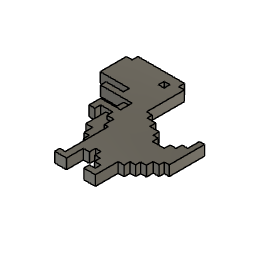
dino (Autodesk Fusion 360 design; units mm, degrees)
Autodesk Fusion 360 part; units mm, degrees
sketch "Dino" plane through (0, 0, 0) normal (0, 0, 1) x (1, 0, 0)
  line L0 (16.5, 0) -> (20, 0)
  line L1 (20, 0) -> (20, 5)
  line L2 (20, 5) -> (21.8166, 5)
  line L3 (21.8166, 5) -> (21.8166, 6.8132)
  line L4 (21.8166, 6.8132) -> (23.4038, 6.8132)
  line L5 (23.4038, 6.8132) -> (23.4038, 5)
  line L6 (23.4038, 5) -> (25, 5)
  line L7 (25, 5) -> (25, 3.315)
  line L8 (25, 3.315) -> (26.8534, 3.315)
  line L9 (26.8534, 3.315) -> (26.8534, 1.6631)
  line L10 (26.8534, 1.6631) -> (25.1529, 1.6631)
  line L11 (25.1529, 1.6631) -> (25.1529, 0)
  line L12 (25.1529, 0) -> (28.5781, 0)
  line L13 (28.5781, 0) -> (28.5781, 6.758)
  line L14 (28.5781, 6.758) -> (30.3565, 6.758)
  line L15 (30.3565, 6.758) -> (30.3565, 8.5127)
  line L16 (30.3565, 8.5127) -> (32, 8.5127)
  line L17 (32, 8.5127) -> (32, 10)
  line L18 (32, 10) -> (33.7351, 10)
  line L19 (33.7351, 10) -> (33.7351, 12)
  line L20 (33.7351, 12) -> (35.5, 12)
  line L21 (35.5, 12) -> (35.5, 13.5)
  line L22 (35.5, 13.5) -> (37, 13.5)
  line L23 (37, 13.5) -> (37, 24)
  line L24 (37, 24) -> (35.5, 24)
  line L25 (35.5, 24) -> (35.5, 20.5)
  line L26 (35.5, 20.5) -> (33.7869, 20.5)
  line L27 (33.7869, 20.5) -> (33.7869, 18.75)
  line L28 (33.7869, 18.75) -> (32, 18.75)
  line L29 (32, 18.75) -> (32, 17.0258)
  line L30 (32, 17.0258) -> (28.5, 17.0258)
  line L31 (28.5, 17.0258) -> (28.5, 18.75)
  line L32 (28.5, 18.75) -> (27, 18.75)
  line L33 (27, 18.75) -> (27, 20.5)
  line L34 (27, 20.5) -> (24.2282, 20.5)
  line L35 (24.2282, 20.5) -> (24.2282, 22.2618)
  line L36 (24.2282, 22.2618) -> (21.6914, 22.2618)
  line L37 (21.6914, 22.2618) -> (21.6914, 23.7839)
  line L38 (21.6914, 23.7839) -> (20, 23.7839)
  line L39 (20, 23.7839) -> (20, 35)
  line L40 (20, 35) -> (18.3225, 35)
  line L41 (18.3225, 35) -> (18.3225, 36.7116)
  line L42 (18.3225, 36.7116) -> (4.5, 36.7116)
  line L43 (4.5, 36.7116) -> (4.5, 35)
  line L44 (4.5, 35) -> (2.7971, 35)
  line L45 (2.7971, 35) -> (2.7971, 27.2137)
  line L46 (2.7971, 27.2137) -> (11.4112, 27.2137)
  line L47 (11.4112, 27.2137) -> (11.4112, 25.5)
  line L48 (11.4112, 25.5) -> (6.2675, 25.5)
  line L49 (6.2675, 25.5) -> (6.2675, 23.8448)
  line L50 (6.2675, 23.8448) -> (13.127, 23.8448)
  line L51 (13.127, 23.8448) -> (13.127, 20.4572)
  line L52 (13.127, 20.4572) -> (9.6973, 20.4572)
  line L53 (9.6973, 20.4572) -> (9.6973, 17)
  line L54 (9.6973, 17) -> (11.4121, 17)
  line L55 (11.4121, 17) -> (11.4121, 18.7286)
  line L56 (11.4121, 18.7286) -> (13, 18.7286)
  line L57 (13, 18.7286) -> (13, 12.7374)
  line L58 (13, 12.7374) -> (15, 12.7374)
  line L59 (15, 12.7374) -> (15, 10.206)
  line L60 (15, 10.206) -> (16.5, 10.206)
  line L61 (16.5, 10.206) -> (16.5, 8.5)
  line L62 (16.5, 8.5) -> (18.1296, 8.5)
  line L63 (18.1296, 8.5) -> (18.1296, 1.5)
  line L64 (18.1296, 1.5) -> (16.5, 1.5)
  line L65 (16.5, 1.5) -> (16.5, 0)
  line L66 (13.127, 23.8448) -> (15.6157, 23.8448)
  line L67 (15.6157, 23.8448) -> (15.6157, 20.4572)
  line L68 (15.6157, 20.4572) -> (13.127, 20.4572)
  line L69 (13, 18.7286) -> (15, 18.7286)
  line L70 (15, 18.7286) -> (15, 17)
  line L71 (15, 17) -> (17, 17)
  line L72 (17, 17) -> (17, 14.1994)
  line L73 (17, 14.1994) -> (18.1296, 14.1994)
  line L74 (18.1296, 14.1994) -> (18.1296, 8.5)
  line L75 (14.802, 34.2204) -> (14.802, 32.5)
  line L76 (14.802, 32.5) -> (16.5, 32.5)
  line L77 (16.5, 32.5) -> (16.5, 34.2204)
  line L78 (16.5, 34.2204) -> (14.802, 34.2204)
  constraint horizontal L0
  constraint perpendicular L0 L1
  constraint perpendicular L1 L2
  constraint perpendicular L0 L3
  constraint perpendicular L3 L4
  constraint perpendicular L0 L5
  constraint perpendicular L3 L6
  constraint perpendicular L0 L7
  constraint perpendicular L7 L8
  constraint perpendicular L8 L9
  constraint perpendicular L9 L10
  constraint perpendicular L8 L11
  constraint perpendicular L9 L12
  constraint perpendicular L12 L13
  constraint perpendicular L13 L14
  constraint perpendicular L14 L15
  constraint perpendicular L15 L16
  constraint perpendicular L16 L17
  constraint perpendicular L15 L18
  constraint perpendicular L18 L19
  constraint perpendicular L19 L20
  constraint perpendicular L20 L21
  constraint perpendicular L19 L22
  constraint perpendicular L22 L23
  constraint perpendicular L23 L24
  constraint perpendicular L22 L25
  constraint perpendicular L23 L26
  constraint perpendicular L26 L27
  constraint perpendicular L27 L28
  constraint perpendicular L26 L29
  constraint perpendicular L27 L30
  constraint perpendicular L30 L31
  constraint perpendicular L31 L32
  constraint perpendicular L32 L33
  constraint perpendicular L31 L34
  constraint perpendicular L34 L35
  constraint perpendicular L35 L36
  constraint perpendicular L36 L37
  constraint perpendicular L37 L38
  constraint perpendicular L36 L39
  constraint perpendicular L37 L40
  constraint perpendicular L40 L41
  constraint perpendicular L41 L42
  constraint perpendicular L42 L43
  constraint perpendicular L43 L44
  constraint perpendicular L42 L45
  constraint perpendicular L45 L46
  constraint perpendicular L46 L47
  constraint perpendicular L45 L48
  constraint perpendicular L48 L49
  constraint perpendicular L49 L50
  constraint perpendicular L50 L51
  constraint perpendicular L51 L52
  constraint perpendicular L52 L53
  constraint perpendicular L53 L54
  constraint perpendicular L54 L55
  constraint perpendicular L55 L56
  constraint perpendicular L52 L57
  constraint perpendicular L57 L58
  constraint perpendicular L58 L59
  constraint perpendicular L59 L60
  constraint perpendicular L60 L61
  constraint perpendicular L61 L62
  constraint perpendicular L60 L63
  constraint perpendicular L63 L64
  constraint perpendicular L64 L65
  constraint perpendicular L51 L66
  constraint perpendicular L50 L67
  constraint perpendicular L67 L68
  constraint perpendicular L57 L69
  constraint perpendicular L56 L70
  constraint perpendicular L70 L71
  constraint perpendicular L71 L72
  constraint perpendicular L72 L73
  constraint perpendicular L62 L74
  constraint vertical L75
  constraint perpendicular L75 L76
  constraint perpendicular L76 L77
  constraint perpendicular L75 L78
extrude "Extrude1" add sketch "Dino" along normal blind 3 contours L0 L1 L2 L3 L4 L5 L6 L7 L8 L9 L10 L11 L12 L13 L14 L15 L16 L17 L18 L19 L20 L21 L22 L23 L24 L25 L26 L27 L28 L29 L30 L31 L32 L33 L34 L35 L36 L37 L38 L39 L40 L41 L42 L43 L44 L45 L46 L47 L48 L49 L50 L52 L53 L54 L55 L56 L63 L64 L65 L66 L67 L68 L69 L70 L71 L72 L73 L74
extrude "Extrude2" add sketch "Dino" along normal blind 2 contours L57 L58 L59 L60 L61 L62 L69 L70 L71 L72 L73 L74 | L51 L66 L67 L68
named bodies: "Dino"
